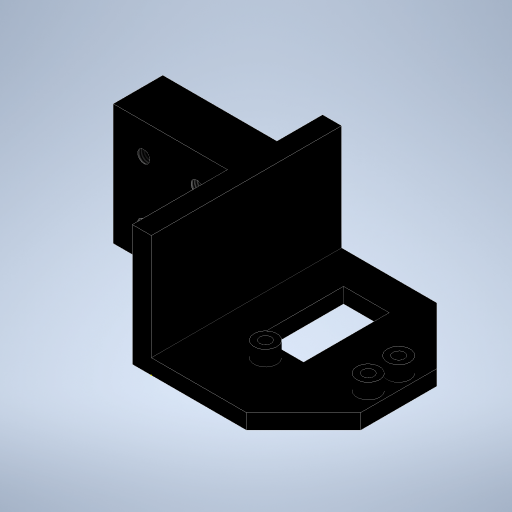
# Autodesk Inventor part: podstawachwytak
Saved by Autodesk Inventor 2024.2 (Build 282272000, 272)
## iProperties
Created: 2023-11-11
Part Number: podstawachwytak
Material: Generic
Document SubType Name: Modeling
Designer: Igor Sarnowski
Density: 1 g/cm^3
Appearance: Default
Author: Igor Sarnowski
Autodesk Inventor part; units mm, degrees
ref_plane "YZ Plane" through (0, 0, 0) normal (1, 0, 0) x (0, 1, 0)
ref_plane "XZ Plane" through (0, 0, 0) normal (0, 1, 0) x (-1, 0, 0)
ref_plane "XY Plane" through (0, 0, 0) normal (0, 0, 1) x (1, 0, 0)
sketch "Sketch1" plane through (0, 0, 0) normal (0, 1, 0) x (-1, 0, 0)
  point P0 (0, 0)
sketch "Sketch2" plane through (0, 0, 0) normal (0, 1, 0) x (-1, 0, 0)
  line L0 (0, 0) -> (0, -50)
  line L1 (0, -50) -> (-25, -50)
  line L2 (-40, -35) -> (-40, -15)
  line L3 (-25, 0) -> (0, 0)
  line L4 (-25, -50) -> (-40, -35)
  line L5 (-25, 0) -> (-40, -15)
  line L6 (-9, -35) -> (-9, -41.5)
  line L7 (-9, -41.5) -> (-21, -41.5)
  line L8 (-21, -41.5) -> (-21, -19)
  line L9 (-21, -19) -> (-9, -19)
  line L10 (-9, -19) -> (-9, -35)
  circle A0 centre (-15, -15) radius 3
  line L11 (0, -25) -> (-40, -25)
  circle A1 centre (-15, -15) radius 1.5
  line L12 (0, 0) -> (5, 0)
  line L13 (5, 0) -> (5, -50)
  line L14 (5, -50) -> (0, -50)
  circle A2 centre (-36, -21) radius 3
  circle A3 centre (-36, -29) radius 3
  circle A4 centre (-36, -21) radius 1.5
  circle A5 centre (-36, -29) radius 1.5
  dimension "d0" = 50
  dimension "d1" = 25
  dimension "d4" = 20
  dimension "d7" = 6.5
  dimension "d8" = 12
  dimension "d9" = 22.5
  dimension "d10" = 6
  dimension "d13" = 3
  dimension "d16" = 5
  dimension "d17" = 6
  dimension "d18" = 6
  dimension "d19" = 3
  dimension "d20" = 3
  constraints: 30 end point, 6 centre point, 6 perpendicular, 3 coincident, 2 midpoint, 1 collinear, 1 horizontal, 1 point on line, 1 vertical
  measures "d0" distance of L0.start L0.end
  measures "d1" distance of L0.end L1.end
  measures "d4" distance of L2.start L2.end
  measures "d7" distance of L6.start L6.end
  measures "d8" distance of L6.end L7.end
  measures "d9" distance of L7.end L8.end
  measures "d10" diameter of A0
  measures "d13" diameter of A1
  measures "d16" distance of L0.start L12.end
  measures "d17" diameter of A2
  measures "d18" diameter of A3
  measures "d19" diameter of A4
  measures "d20" diameter of A5
extrude "Extrusion1" add sketch "Sketch2" along normal blind 8 contours A0 | A2 | A3
extrude "Extrusion2" add sketch "Sketch2" along normal blind 4 contours L0 L11 L10 L9 L8 L2 L5 L3 | L0 L1 L4 L2 L11 L8 L7 L6 L10
extrude "Extrusion3" add sketch "Sketch2" along normal blind 31.807 contours L12 L13 L14 L0
sketch "Szkic4" plane through (-5, 0, -50) normal (-1, 0, 0) x (0, 0, 1)
  line L0 (0, 0) -> (50, 0) projected
  line L1 (50, 0) -> (50, 31.807) projected
  line L2 (0, 31.807) -> (50, 31.807) projected
  line L3 (0, 0) -> (0, 31.807) projected
  line L4 (38, 21.6151) -> (12, 21.6151)
  line L5 (25, 21.6151) -> (25, 0)
  line L6 (25, 21.6151) -> (25, 31.807)
  line L7 (12, 21.6151) -> (12, 31.807)
  line L8 (12, 21.6151) -> (12, 0)
  dimension "d32" = 31.807
  dimension "d33" = 50
  dimension "d34" = 26
  dimension "d35" = 12
  dimension "d36" = 12
  dimension "d37" = 13
  constraints: 10 end point, 3 midpoint, 3 point on line, 1 horizontal, 1 perpendicular
  measures "d32" distance of L0.end L1.end
  measures "d33" distance of L2.start L1.end
  measures "d34" distance of L4.start L4.end
  measures "d35" distance from line of L3 L4.end
  measures "d36" distance from line of L1 L4.start
  measures "d37" distance of L4.end L5.start
extrude "Wyciągnięcie proste5" add sketch "Szkic4" along normal blind 30 contours L8 L4 L5 L0 | L7 L2 L6 L4
sketch "Szkic5" plane through (-5, 0, -38) normal (0, 0, -1) x (-1, 0, 0)
  line L0 (0, 0) -> (30, 0) projected
  line L1 (0, 31.807) -> (30, 31.807) projected
  line L2 (30, 31.807) -> (30, 0) projected
  line L3 (0, 0) -> (0, 31.807) projected
  line L4 (0, 0) -> (30, 0) projected
  line L5 (30, 31.807) -> (30, 0) projected
  line L6 (0, 31.807) -> (30, 31.807) projected
  point P0 (-5, 0)
  point P1 (22, 8)
  point P2 (22, 23.807)
  point P3 (8, 8)
  point P4 (8, 23.807)
  dimension "d40" = 8
  dimension "d41" = 8
  dimension "d42" = 8
  dimension "d43" = 8
  dimension "d51" = 8
  dimension "d52" = 8
  dimension "d53" = 8
  dimension "d54" = 8
  measures "d40" distance from line of L0 point (22, 8)
  measures "d41" distance from line of L1 point (22, 23.807)
  measures "d42" distance from line of L2 point (22, 23.807)
  measures "d43" distance from line of L2 point (22, 8)
  measures "d51" distance from line of L0 point (8, 8)
  measures "d52" distance from line of L1 point (8, 23.807)
  measures "d53" distance from line of L3 point (8, 23.807)
  measures "d54" distance from line of L3 point (8, 8)
hole "Otwór1" at (-27, 8, -38) at (-27, 23.807, -38) at (-13, 8, -38) at (-13, 23.807, -38) direction (0, 0, 1) diameter 3.242 end through all thread size "M4x0.7" designation "M4" class "6H" standard "GB Metric profile"
sketch "Szkic6" plane through (-5, 0, -38) normal (0, 0, -1) x (-1, 0, 0)
  circle A0 centre (8, 23.807) radius 1.621 projected
  circle A1 centre (8, 8) radius 1.621 projected
  circle A2 centre (22, 23.807) radius 1.621 projected
  circle A3 centre (22, 8) radius 1.621 projected
  line L0 (0, 0) -> (0, 31.807) projected
  line L1 (0, 0) -> (30, 0) projected
  line L2 (30, 31.807) -> (30, 0) projected
  line L3 (0, 31.807) -> (30, 31.807) projected
  circle A4 centre (8, 23.807) radius 4
  circle A5 centre (22, 23.807) radius 4
  circle A6 centre (22, 8) radius 4
  circle A7 centre (8, 8) radius 4
  point P0 (-5, 0)
  dimension "d55" = 8
  dimension "d56" = 8
  dimension "d57" = 8
  dimension "d58" = 8
  constraints: 4 centre point, 4 coincident
  measures "d55" diameter of A4
  measures "d56" diameter of A5
  measures "d57" diameter of A6
  measures "d58" diameter of A7
extrude "Wyciągnięcie proste6" cut sketch "Szkic6" against normal blind 9 contours A4 | A5 | A6 | A7
body "Solid1"
